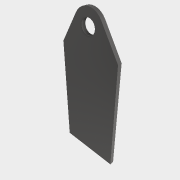
# Autodesk Inventor part: Skid Lifting Plate
Saved by Autodesk Inventor 2019.1 (Build 231200000, 200)
## iProperties
Created: 2018-08-31
Part Number: Skid Lifting Plate
Material: Steel, Galvanized
Document SubType Name: Modeling
Designer: alid
Density: 7.85 g/cm^3
Appearance: Galvanized
Description: Skid Lifting Plate
Stock Number: NA
Mass: 3810.54 g
Surface Area: 1075.86 cm^2
Volume: 485.419 cm^3
Author: alid
Title: Manufactured Part
Revision Number: A
Autodesk Inventor part; units mm, degrees
ref_plane "YZ Plane" through (0, 0, 0) normal (1, 0, 0) x (0, 1, 0)
ref_plane "XZ Plane" through (0, 0, 0) normal (0, 1, 0) x (-1, 0, 0)
ref_plane "XY Plane" through (0, 0, 0) normal (0, 0, 1) x (1, 0, 0)
sketch "Sketch1" plane through (0, 0, 0) normal (0, 1, 0) x (-1, 0, 0)
  line L0 (-75, 0) -> (75, 0)
  line L1 (75, 0) -> (75, 275)
  line L2 (75, 275) -> (-75, 275) construction
  line L3 (-75, 275) -> (-75, 0)
  circle A0 centre (0, 325) radius 37.5
  line L4 (-75, 275) -> (-31.8965, 344.7197)
  line L5 (75, 275) -> (31.8965, 344.7197)
  point P0 (0, 0)
  point P1 (0, 0)
  dimension "d2" = 75
  dimension "d3" = 50
  constraints: 12 end point, 2 parallel, 2 point on circle, 2 tangent, 2 vertical alignment, 1 centre point, 1 coincident, 1 horizontal, 1 horizontal alignment, 1 midpoint, 1 perpendicular
  measures "d2" diameter of A0
  measures "d3" distance from line of L2 A0.centre
extrude "Extrusion1" add sketch "Sketch1" along normal blind 10
sketch "Sketch2" plane through (0, 0, 0) normal (0, -1, 0) x (1, 0, 0)
  arc A0 (31.8965, 344.7197) -> (-31.8965, 344.7197) centre (0, 325) ccw projected
  point P0 (0, 0)
  constraints: 1 coincident
hole "Hole1" at (0, 0, 325) direction (0, 1, 0) diameter 35 end through all
sketch "Sketch3" plane through (-75, 0, 0) normal (-1, 0, 0) x (0, 0, 1)
  line L0 (11, 10) -> (11, 54)
  line L1 (11, 54) -> (41, 84)
  line L2 (41, 84) -> (159, 84)
  line L3 (159, 84) -> (189, 54)
  line L4 (189, 54) -> (189, 10)
  line L5 (0, 10) -> (275, 10) projected
  line L6 (189, 10) -> (11, 10)
  dimension "d14" = 135
  dimension "d18" = 11
  dimension "d19" = 74
  dimension "d20" = 30
  dimension "d22" = 178
  dimension "d26" = 21
  constraints: 4 end point, 2 point on line, 1 horizontal alignment
  measures "d26" distance of point (-75, -189) L6.end
sketch "Sketch6" plane through (-75, 10, 210) normal (0, 0, 1) x (1, 0, 0)
  line L0 (0, 0) -> (10, 0)
  line L1 (10, 0) -> (10, 25)
  line L2 (10, 25) -> (0, 25)
  line L3 (0, 25) -> (0, 0)
  point P0 (75, -10)
  dimension "d27" = 10
  dimension "d28" = 25
  constraints: 8 end point, 2 parallel, 1 horizontal, 1 perpendicular
  measures "d27" distance of L2.end L1.end
  measures "d28" distance of L1.end L0.end
sketch3d "3D Sketch1"
sketch "Sketch7" plane through (0, 10, 0) normal (0, 1, 0) x (1, 0, 0)
  circle A0 centre (0, -325) radius 17.5 projected
  circle A1 centre (0, -325) radius 27.5
  point P0 (0, 0)
  dimension "d31" = 10
  constraints: 1 centre point, 1 coincident
  measures "d31" radial gap between concentric circles of A1 A0
sketch "Sketch8" plane through (-75, 35, 210) normal (0, 1, 0) x (1, 0, 0)
  line L0 (0, -65) -> (43.1035, -134.7197) projected
  arc A0 (43.1035, -134.7197) -> (106.8965, -134.7197) centre (75, -115) ccw projected
  line L1 (106.8965, -134.7197) -> (150, -65) projected
  line L2 (150, -65) -> (150, 0) projected
  line L3 (140, 0) -> (150, 0) projected
  line L4 (140, -62.1584) -> (140, 0) projected
  line L5 (98.3907, -129.4611) -> (140, -62.1584) projected
  arc A1 (51.6093, -129.4611) -> (98.3907, -129.4611) centre (75, -115) ccw projected
  line L6 (10, -62.1584) -> (51.6093, -129.4611) projected
  line L7 (10, 0) -> (10, -62.1584) projected
  line L8 (10, 0) -> (0, 0) projected
  line L9 (0, 0) -> (0, -65) projected
  line L10 (140, 0) -> (10, 0)
  circle A2 centre (75, -115) radius 17.5 projected
  point P0 (75, 210)
  constraints: 2 end point, 1 horizontal
body "Solid1"
body "Solid2"
body "Solid3"
body "Solid4"
body "Solid5"
